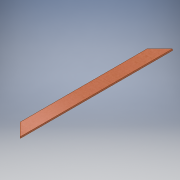
# Autodesk Inventor part: EdgeCover
Saved by Autodesk Inventor 2019.3 (Build 233278000, 278)
## iProperties
Created: 2019-01-19
Part Number: EdgeCover
Material: Holz (Walnuss)
Document SubType Name: Modeling
Designer: Jonas
Density: 0.55 g/cm^3
Appearance: Walnuss - natur - poliert
Author: Jonas
Autodesk Inventor part; units mm, degrees
ref_plane "YZ Plane" through (0, 0, 0) normal (1, 0, 0) x (0, 1, 0)
ref_plane "XZ Plane" through (0, 0, 0) normal (0, 1, 0) x (-1, 0, 0)
ref_plane "XY Plane" through (0, 0, 0) normal (0, 0, 1) x (1, 0, 0)
sketch "Skizze1" plane through (0, 0, 0) normal (0, 1, 0) x (-1, 0, 0)
  line L0 (12.5, 125) -> (12.5, -125)
  line L1 (-12.5, -150) -> (-12.5, 150)
  line L2 (-12.5, 150) -> (10.5769, -126.9231) construction
  line L3 (12.5, 150) -> (-12.5, -150) construction
  line L4 (-12.5, 150) -> (12.5, 125)
  line L5 (-12.5, -150) -> (12.5, -125)
  point P0 (0, 0)
  dimension "d5" = 45
  dimension "d7" = 45
  dimension "d8" = 300
  dimension "d9" = 25
  constraints: 12 end point, 2 point on line, 1 midpoint, 1 parallel
  measures "d5" angle of L1 L4
  measures "d7" angle of L1 L5
  measures "d8" distance of L1.start L1.end
  measures "d9" distance between parallel lines of L0 L1
extrude "Extrusion1" add sketch "Skizze1" along normal blind 3
